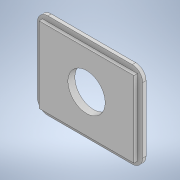
# Autodesk Inventor part: screen-dc-port-front
Saved by Autodesk Inventor 2020 (Build 240168000, 168)
## iProperties
Created: 2019-08-07
Part Number: screen-dc-port-front
Material: Generic
Document SubType Name: Modeling
Designer: Senior Design
Density: 1 g/cm^3
Appearance: Default
Author: Senior Design
Autodesk Inventor part; units mm, degrees
ref_plane "YZ Plane" through (0, 0, 0) normal (1, 0, 0) x (0, 1, 0)
ref_plane "XZ Plane" through (0, 0, 0) normal (0, 1, 0) x (-1, 0, 0)
ref_plane "XY Plane" through (0, 0, 0) normal (0, 0, 1) x (1, 0, 0)
sketch "Sketch1" plane through (0, 0, 0) normal (0, 0, 1) x (1, 0, 0)
  line L0 (13.75, -11) -> (-13.75, -11)
  line L1 (-13.75, -11) -> (-13.75, 11)
  line L2 (-13.75, 11) -> (13.75, 11)
  line L3 (13.75, 11) -> (13.75, -11)
  line L4 (13.75, -11) -> (-13.75, 11) construction
  line L5 (-13.75, -11) -> (13.75, 11) construction
  circle A0 centre (0, 0) radius 5.4
  dimension "d0" = 27.5
  dimension "d1" = 22
  dimension "d2" = 10.8
  constraints: 12 end point, 2 midpoint, 2 parallel, 1 centre point, 1 coincident, 1 horizontal, 1 perpendicular
  measures "d0" distance of L0.start L0.end
  measures "d1" distance of L0.end L1.end
  measures "d2" diameter of A0
extrude "Extrusion1" add sketch "Sketch1" along normal blind 1
sketch "Sketch2" plane through (0, 0, 0) normal (0, 0, -1) x (-1, 0, 0)
  line L0 (15.25, 12.5) -> (-15.25, 12.5)
  line L1 (-15.25, 12.5) -> (-15.25, -12.5)
  line L2 (-15.25, -12.5) -> (15.25, -12.5)
  line L3 (15.25, -12.5) -> (15.25, 12.5)
  line L4 (15.25, 12.5) -> (-15.25, -12.5) construction
  line L5 (-15.25, 12.5) -> (15.25, -12.5) construction
  line L6 (-13.75, -11) -> (-13.75, 11) projected
  line L7 (-13.75, 11) -> (13.75, 11) projected
  circle A0 centre (0, 0) radius 5.4
  circle A1 centre (0, 0) radius 5.4 projected
  dimension "d5" = 1.5
  dimension "d6" = 1.5
  constraints: 12 end point, 2 midpoint, 2 parallel, 2 perpendicular, 1 centre point, 1 coincident, 1 concentric
  measures "d5" distance between parallel lines of L6 L1
  measures "d6" distance between parallel lines of L0 L7
extrude "Extrusion2" add sketch "Sketch2" along normal blind 1
fillet "Fillet1" radius 3 4 edges at (-15.25, 12.5, -0.5) (-15.25, -12.5, -0.5) (15.25, -12.5, -0.5) (15.25, 12.5, -0.5)
body "Solid1"
